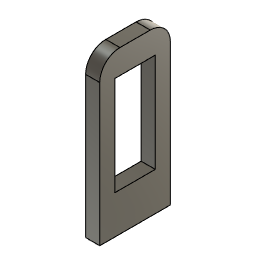
Previsagra v2 v7 (Autodesk Fusion 360 design; units mm, degrees)
Autodesk Fusion 360 part; units mm, degrees
note: some values were not read from the file. Set by a fixed rule: which sketch regions a step uses.
sketch "Boceto1" plane through (0, 0, 0) normal (1, 0, 0) x (0, 1, 0)
  line L0 (45, 15) -> (45, 70)
  line L1 (80, 15) -> (80, 70)
  arc A0 (80, 70) -> (70, 80) centre (70, 70) ccw
  arc A1 (55, 80) -> (45, 70) centre (55, 70) ccw
  line L2 (55, 80) -> (70, 80)
  line L3 (72.5, 19) -> (72.5, 68)
  line L4 (52.5, 68) -> (52.5, 19)
  line L5 (45, 15) -> (45, 0)
  line L6 (45, 0) -> (80, 0)
  line L7 (80, 0) -> (80, 15)
  line L8 (52.5, 68) -> (72.5, 68)
  line L9 (52.5, 19) -> (72.5, 19)
  constraint tangent A0 L2
  constraint parallel L0 L5
  constraint perpendicular L1 L6
  constraint perpendicular L6 L7
  constraint perpendicular L3 L8
  constraint perpendicular L3 L9
extrude "Extruir2" add sketch "Boceto1" along normal blind 7 makes body 1
copy_body "Cuerpo - > Comp.1" bodies 1 removing the originals makes body 2 in component "Component"
scale "Escala1" factor 2 about (0, 55, 80) bodies 2 in component "Component"
scale "Escala2" factor 0.5 about (14, 50, 56) bodies 2 in component "Component"
component "Component" placed x (1, 0, 0) y (0, 1, 0) z (0, 0, 1) at (0, 0, 0)
